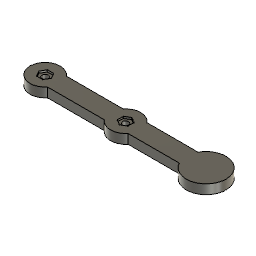
Female to servo (Autodesk Fusion 360 design; units mm, degrees)
part number: 2025-11-19-16-47-52-691
part number: 2025-11-19-16-48-20-946
Autodesk Fusion 360 part; units mm, degrees
note: some values were not read from the file. Chosen so that the rebuilt part matches the saved one: which face or edge a step refers to. Set by a fixed rule: which sketch regions a step uses.
sketch "body_90" plane through (0, 0, 0) normal (0, 0, 1) x (1, 0, 0) in component "sciccor arm right size"
sketch "Sketch2" plane through (0, 0, 0) normal (0, 0, 1) x (1, 0, 0) in component "sciccor arm right size"
sketch "Sketch3" plane through (0, 0, 0) normal (0, 0, 1) x (1, 0, 0) in component "sciccor arm right size"
  circle A0 centre (0, 5) radius 5
  circle A1 centre (42.5, 5) radius 5
  circle A2 centre (85, 5) radius 5
  line L0 (36.255, 10) -> (6.245, 10)
  line L1 (6.245, 0) -> (36.255, 0)
  line L2 (48.745, 0) -> (78.755, 0)
  line L3 (78.755, 10) -> (48.745, 10)
  arc A3 (78.755, 0) -> (78.755, 10) centre (85, 5) ccw
  arc A4 (48.745, 10) -> (36.255, 10) centre (42.5, 5) ccw
  arc A5 (36.255, 0) -> (48.745, 0) centre (42.5, 5) ccw
  arc A6 (6.245, 10) -> (6.245, 0) centre (0, 5) ccw
  line L4 (3.2909, 5.0119) -> (1.6351, 7.8559)
  line L5 (1.6351, 7.8559) -> (-1.6558, 7.844)
  line L6 (-1.6558, 7.844) -> (-3.2909, 4.9881)
  line L7 (-3.2909, 4.9881) -> (-1.6351, 2.1441)
  line L8 (-1.6351, 2.1441) -> (1.6558, 2.156)
  line L9 (1.6558, 2.156) -> (3.2909, 5.0119)
  line L10 (45.35, 6.6454) -> (42.5, 8.2909)
  line L11 (42.5, 8.2909) -> (39.65, 6.6454)
  line L12 (39.65, 6.6454) -> (39.65, 3.3546)
  line L13 (39.65, 3.3546) -> (42.5, 1.7091)
  line L14 (42.5, 1.7091) -> (45.35, 3.3546)
  line L15 (45.35, 3.3546) -> (45.35, 6.6454)
  line L16 (87.85, 6.6454) -> (85, 8.2909)
  line L17 (85, 8.2909) -> (82.15, 6.6454)
  line L18 (82.15, 6.6454) -> (82.15, 3.3546)
  line L19 (82.15, 3.3546) -> (85, 1.7091)
  line L20 (85, 1.7091) -> (87.85, 3.3546)
  line L21 (87.85, 3.3546) -> (87.85, 6.6454)
  circle A7 centre (0, 5) radius 1.6
  circle A8 centre (42.5, 5) radius 1.6
  circle A9 centre (85, 5) radius 1.6
  point P0 (0, 5)
  point P1 (42.5, 5)
  point P2 (85, 5)
  dimension "d25" = 16
  dimension "d27" = 16
  dimension "d30" = 16
  dimension "d31" = 10
  dimension "d32" = 10
  dimension "d33" = 10
  dimension "d34" = 2.85
  dimension "d35" = 2.85
  dimension "d36" = 2.85
  dimension "d46" = 3.2
  dimension "d47" = 3.2
  dimension "d48" = 3.2
  constraint concentric A0 A6
  constraint concentric A1 A4
  constraint concentric A2 A3
  constraint coincident L1.end A4
  constraint concentric A4 A5
  constraint coincident P0 A0.centre
  constraint coincident P1 A1.centre
  constraint coincident P2 A2.centre
  constraint concentric A6 A7
  constraint concentric A1 A8
  constraint concentric A3 A9
  measures "d25" diameter of A4
  measures "d27" diameter of A3
  measures "d30" diameter of A6
  measures "d31" diameter of A0
  measures "d32" diameter of A1
  measures "d33" diameter of A2
  measures "d34" distance of P0 L9
  measures "d35" distance of P1 L15
  measures "d36" distance of P2 L21
  measures "d46" diameter of A7
  measures "d47" diameter of A8
  measures "d48" diameter of A9
extrude "Extrude1" add sketch "Sketch3" along normal blind 5 contours A0 | A1 | A2 | L0 L1 L2 L3 A3 A4 A5 A6 makes body 1 in component "sciccor arm right size"
extrude "Extrude2" add sketch "Sketch3" along normal blind 4 contours L4 L5 L6 L7 L8 L9 | L10 L11 L12 L13 L14 L15 | L16 L17 L18 L19 L20 L21 | A7 | A8 | A9 bodies 1 in component "sciccor arm right size"
extrude "Extrude1'" add sketch "Sketch3" along normal blind 5 separate body contours A0 | A1 | A2 | L0 L1 L2 L3 A3 A4 A5 A6 makes body 2
extrude "Extrude2'" add sketch "Sketch3" along normal blind 4 contours L4 L5 L6 L7 L8 L9 | L10 L11 L12 L13 L14 L15 | L16 L17 L18 L19 L20 L21 bodies 2
sketch "Sketch1" plane through (0, 0, 0) normal (0, 0, 1) x (1, 0, 0)
sketch "Sketch2 (2)" plane through (0, 0, 0) normal (0, 0, 1) x (1, 0, 0)
  circle A0 centre (85, 5) radius 10.5
  dimension "d59" = 21
  measures "d59" diameter of A0
extrude "Extrude6" add sketch "Sketch2 (2)" along normal blind 5 bodies 2
sketch "Sketch3 (2)" plane through (0, 0, 0) normal (0, 0, -1) x (1, 0, 0)
  arc A0 (75.7669, -10) -> (75.7669, 0) centre (85, -5) ccw
  line L0 (75.7669, 0) -> (48.745, 0)
  arc A1 (48.745, 0) -> (36.255, 0) centre (42.5, -5) ccw
  line L1 (36.255, 0) -> (6.245, 0)
  arc A2 (6.245, 0) -> (6.245, -10) centre (0, -5) ccw
  line L2 (6.245, -10) -> (36.255, -10)
  arc A3 (36.255, -10) -> (48.745, -10) centre (42.5, -5) ccw
  line L3 (48.745, -10) -> (75.7669, -10)
  circle A4 centre (0, -5) radius 1.6
  circle A5 centre (42.5, -5) radius 1.6
  circle A6 centre (85, -5) radius 10.5
  constraint concentric A0 A6
extrude "Extrude7" add sketch "Sketch3 (2)" against normal blind 1 contours A0 A6 bodies 2
sketch "Sketch4" plane through (0, 0, -6) normal (0, 0, -1) x (1, 0, 0)
  circle A0 centre (85, -5) radius 1.6
  circle A1 centre (85, 3) radius 0.5
  circle A2 centre (85, -13) radius 0.5
  line L0 (87.85, -6.6454) -> (87.85, -3.3546)
  line L1 (87.85, -3.3546) -> (85, -1.7091)
  line L2 (85, -1.7091) -> (82.15, -3.3546)
  line L3 (82.15, -3.3546) -> (82.15, -6.6454)
  line L4 (82.15, -6.6454) -> (85, -8.2909)
  line L5 (85, -8.2909) -> (87.85, -6.6454)
  dimension "d64" = 1
  dimension "d65" = 1
  measures "d64" diameter of A1
  measures "d65" diameter of A2
extrude "Extrude8" cut sketch "Sketch4" against normal blind 5 contours A1 | A2 bodies 2
sketch "Sketch5" plane through (0, 0, 5) normal (0, 0, 1) x (-1, 0, 0)
  line L0 (-75.7669, -10) -> (-48.745, -10)
  arc A0 (-48.745, -10) -> (-36.255, -10) centre (-42.5, -5) ccw
  line L1 (-36.255, -10) -> (-6.245, -10)
  arc A1 (-6.245, -10) -> (-6.245, 0) centre (0, -5) ccw
  line L2 (-6.245, 0) -> (-36.255, 0)
  arc A2 (-36.255, 0) -> (-48.745, 0) centre (-42.5, -5) ccw
  line L3 (-48.745, 0) -> (-75.7669, 0)
  arc A3 (-75.7669, 0) -> (-75.7669, -10) centre (-85, -5) ccw
  line L4 (-3.2909, -5.0119) -> (-1.6558, -2.156)
  line L5 (-1.6558, -2.156) -> (1.6351, -2.1441)
  line L6 (1.6351, -2.1441) -> (3.2909, -4.9881)
  line L7 (3.2909, -4.9881) -> (1.6558, -7.844)
  line L8 (1.6558, -7.844) -> (-1.6351, -7.8559)
  line L9 (-1.6351, -7.8559) -> (-3.2909, -5.0119)
  line L10 (-45.35, -6.6454) -> (-45.35, -3.3546)
  line L11 (-45.35, -3.3546) -> (-42.5, -1.7091)
  line L12 (-42.5, -1.7091) -> (-39.65, -3.3546)
  line L13 (-39.65, -3.3546) -> (-39.65, -6.6454)
  line L14 (-39.65, -6.6454) -> (-42.5, -8.2909)
  line L15 (-42.5, -8.2909) -> (-45.35, -6.6454)
  circle A4 centre (-85, -13) radius 1
  circle A5 centre (-85, 3) radius 1
  dimension "d68" = 2
  dimension "d69" = 2
  measures "d68" diameter of A4
  measures "d69" diameter of A5
extrude "Extrude9" [suppressed]
component "sciccor arm right size" placed x (1, 0, 0) y (0, 1, 0) z (0, 0, 1) at (0, 0, 0)
